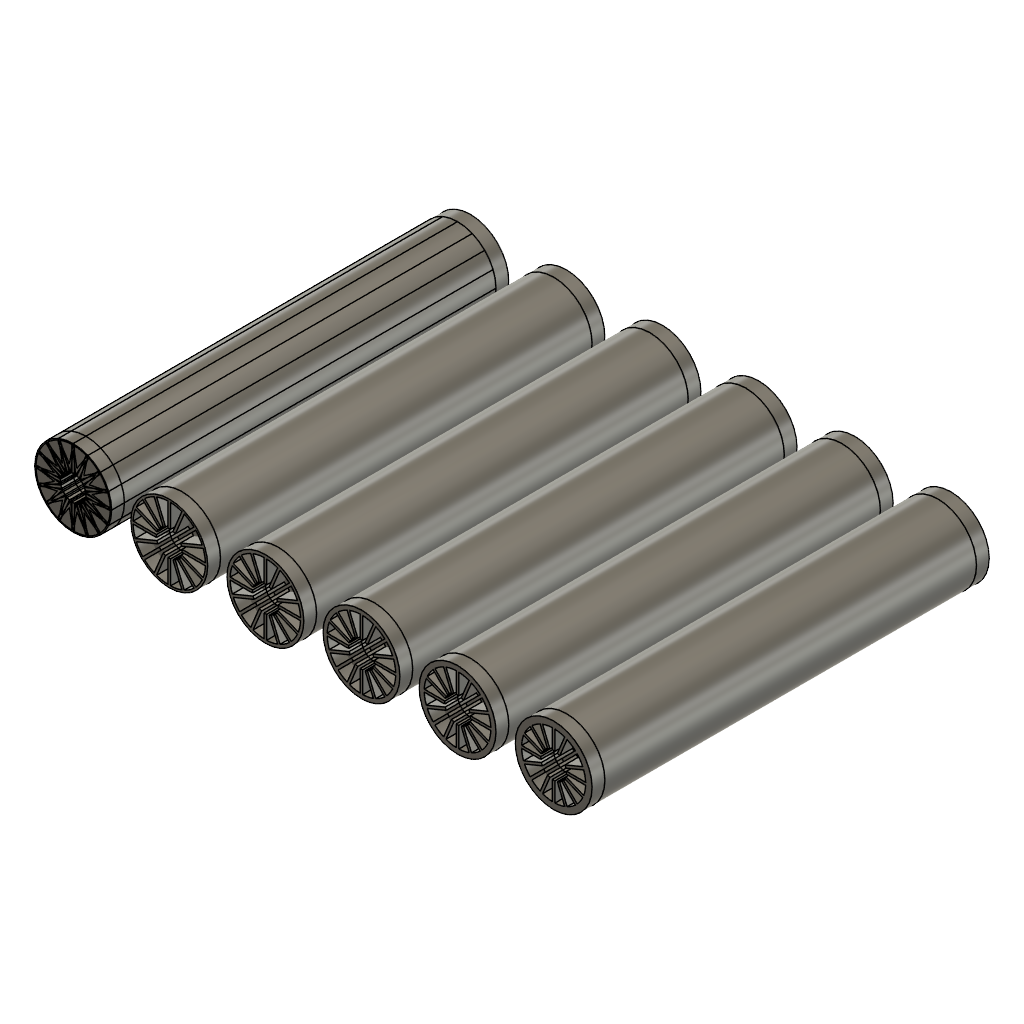
PAMcIA (Autodesk Fusion 360 design; units mm, degrees)
part number: 2026-09-20-16-45-00-598
Autodesk Fusion 360 part; units mm, degrees
sketch "Boceto1" plane through (0, 0, 0) normal (0, 0, 1) x (1, 0, 0)
  line L0 (6, 0) -> (2.9424, 0.5853)
  line L1 (2.9424, 0.5853) -> (5.5433, 2.2961)
  line L2 (5.5433, 2.2961) -> (2.4944, 1.6667)
  line L3 (2.4944, 1.6667) -> (4.2426, 4.2426)
  line L4 (4.2426, 4.2426) -> (1.6667, 2.4944)
  line L5 (1.6667, 2.4944) -> (2.2961, 5.5433)
  line L6 (2.2961, 5.5433) -> (0.5853, 2.9424)
  line L7 (0.5853, 2.9424) -> (0, 6)
  line L8 (0, 6) -> (-0.5853, 2.9424)
  line L9 (-0.5853, 2.9424) -> (-2.2961, 5.5433)
  line L10 (-2.2961, 5.5433) -> (-1.6667, 2.4944)
  line L11 (-1.6667, 2.4944) -> (-4.2426, 4.2426)
  line L12 (-4.2426, 4.2426) -> (-2.4944, 1.6667)
  line L13 (-2.4944, 1.6667) -> (-5.5433, 2.2961)
  line L14 (-5.5433, 2.2961) -> (-2.9424, 0.5853)
  line L15 (-2.9424, 0.5853) -> (-6, 0)
  line L16 (-6, 0) -> (-2.9424, -0.5853)
  line L17 (-2.9424, -0.5853) -> (-5.5433, -2.2961)
  line L18 (-5.5433, -2.2961) -> (-2.4944, -1.6667)
  line L19 (-2.4944, -1.6667) -> (-4.2426, -4.2426)
  line L20 (-4.2426, -4.2426) -> (-1.6667, -2.4944)
  line L21 (-1.6667, -2.4944) -> (-2.2961, -5.5433)
  line L22 (-2.2961, -5.5433) -> (-0.5853, -2.9424)
  line L23 (-0.5853, -2.9424) -> (0, -6)
  line L24 (0, -6) -> (0.5853, -2.9424)
  line L25 (0.5853, -2.9424) -> (2.2961, -5.5433)
  line L26 (2.2961, -5.5433) -> (1.6667, -2.4944)
  line L27 (1.6667, -2.4944) -> (4.2426, -4.2426)
  line L28 (4.2426, -4.2426) -> (2.4944, -1.6667)
  line L29 (2.4944, -1.6667) -> (5.5433, -2.2961)
  line L30 (5.5433, -2.2961) -> (2.9424, -0.5853)
  line L31 (2.9424, -0.5853) -> (6, 0)
  circle A0 centre (0, 0) radius 2
extrude "Extruir1" add sketch "Boceto1" along normal blind 60 makes body 1
sketch "Boceto2" plane through (0, 0, 0) normal (0, 0, 1) x (1, 0, 0)
  circle A0 centre (0, 0) radius 6
  line L0 (5, 0) -> (1.9616, 0.3902)
  line L1 (1.9616, 0.3902) -> (4.6194, 1.9134)
  line L2 (4.6194, 1.9134) -> (1.6629, 1.1111)
  line L3 (1.6629, 1.1111) -> (3.5355, 3.5355)
  line L4 (3.5355, 3.5355) -> (1.1111, 1.6629)
  line L5 (1.1111, 1.6629) -> (1.9134, 4.6194)
  line L6 (1.9134, 4.6194) -> (0.3902, 1.9616)
  line L7 (0.3902, 1.9616) -> (0, 5)
  line L8 (0, 5) -> (-0.3902, 1.9616)
  line L9 (-0.3902, 1.9616) -> (-1.9134, 4.6194)
  line L10 (-1.9134, 4.6194) -> (-1.1111, 1.6629)
  line L11 (-1.1111, 1.6629) -> (-3.5355, 3.5355)
  line L12 (-3.5355, 3.5355) -> (-1.6629, 1.1111)
  line L13 (-1.6629, 1.1111) -> (-4.6194, 1.9134)
  line L14 (-4.6194, 1.9134) -> (-1.9616, 0.3902)
  line L15 (-1.9616, 0.3902) -> (-5, 0)
  line L16 (-5, 0) -> (-1.9616, -0.3902)
  line L17 (-1.9616, -0.3902) -> (-4.6194, -1.9134)
  line L18 (-4.6194, -1.9134) -> (-1.6629, -1.1111)
  line L19 (-1.6629, -1.1111) -> (-3.5355, -3.5355)
  line L20 (-3.5355, -3.5355) -> (-1.1111, -1.6629)
  line L21 (-1.1111, -1.6629) -> (-1.9134, -4.6194)
  line L22 (-1.9134, -4.6194) -> (-0.3902, -1.9616)
  line L23 (-0.3902, -1.9616) -> (0, -5)
  line L24 (0, -5) -> (0.3902, -1.9616)
  line L25 (0.3902, -1.9616) -> (1.9134, -4.6194)
  line L26 (1.9134, -4.6194) -> (1.1111, -1.6629)
  line L27 (1.1111, -1.6629) -> (3.5355, -3.5355)
  line L28 (3.5355, -3.5355) -> (1.6629, -1.1111)
  line L29 (1.6629, -1.1111) -> (4.6194, -1.9134)
  line L30 (4.6194, -1.9134) -> (1.9616, -0.3902)
  line L31 (1.9616, -0.3902) -> (5, 0)
extrude "Extruir2" add sketch "Boceto2" along normal blind 60 separate body makes body 2
sketch "Boceto3" plane through (0, 0, 0) normal (0, 0, 1) x (1, 0, 0)
  circle A0 centre (0, 0) radius 6
  circle A1 centre (0, 0) radius 5.8
extrude "Extruir3" add sketch "Boceto3" along normal blind 60 separate body makes body 3
sketch "Boceto4" plane through (0, 0, 0) normal (0, 0, 1) x (1, 0, 0)
  line L0 (2, -0.2) -> (5.8, -0.2)
  line L1 (5.8, -0.2) -> (5.8, 0.2)
  line L2 (5.8, 0.2) -> (2, 0.2)
  line L3 (2, 0.2) -> (2, -0.2)
extrude "Extruir4" add sketch "Boceto4" along normal blind 60 separate body makes body 4
pattern_circular "Patrón C1" count 16 over 360 about axis through (0, 0, 1.75) along (0, 0, 1) of bodies 4 makes body 5 at (4.1117, 1.9196, 20) makes body 6 at (3.0641, 3.347, 20) makes body 7 at (1.5501, 4.2648, 20) makes body 8 at (-0.2, 4.5333, 20) makes body 9 at (-1.9196, 4.1117, 20) makes body 10 at (-3.347, 3.0641, 20) makes body 11 at (-4.2648, 1.5501, 20) makes body 12 at (-4.5333, -0.2, 20) makes body 13 at (-4.1117, -1.9196, 20) makes body 14 at (-3.0641, -3.347, 20) makes body 15 at (-1.5501, -4.2648, 20) makes body 16 at (0.2, -4.5333, 20) makes body 17 at (1.9196, -4.1117, 20) makes body 18 at (3.347, -3.0641, 20) makes body 19 at (4.2648, -1.5501, 20)
combine "Combinar1" operation add target body 3 tool bodies 4 5 6 7 8 9 10 11 12 13 14 15 16 17 18 19 4
sketch "Boceto5" plane through (0, 0, 0) normal (0, 0, 1) x (1, 0, 0)
  circle A0 centre (0, 0) radius 6
  circle A1 centre (0, 0) radius 5.65
extrude "Extruir5" add sketch "Boceto5" along normal blind 60 separate body makes body 20
sketch "Boceto6" plane through (0, 0, 0) normal (0, 0, 1) x (1, 0, 0)
  line L0 (2, -0.2) -> (5.65, -0.2)
  line L1 (5.65, -0.2) -> (5.65, 0.2)
  line L2 (5.65, 0.2) -> (2, 0.2)
  line L3 (2, 0.2) -> (2, -0.2)
extrude "Extruir6" add sketch "Boceto6" along normal blind 60 separate body makes body 21
pattern_circular "Patrón C2" count 16 over 360 about axis through (0, 0, 1.75) along (0, 0, 1) of bodies 21 makes body 22 at (4.0193, 1.8813, 20) makes body 23 at (2.9934, 3.2763, 20) makes body 24 at (1.5118, 4.1724, 20) makes body 25 at (-0.2, 4.4333, 40) makes body 26 at (-1.8813, 4.0193, 20) makes body 27 at (-3.2763, 2.9934, 40) makes body 28 at (-4.1724, 1.5118, 20) makes body 29 at (-4.4333, -0.2, 40) makes body 30 at (-4.0193, -1.8813, 20) makes body 31 at (-2.9934, -3.2763, 20) makes body 32 at (-1.5118, -4.1724, 20) makes body 33 at (0.2, -4.4333, 40) makes body 34 at (1.8813, -4.0193, 20) makes body 35 at (3.2763, -2.9934, 20) makes body 36 at (4.1724, -1.5118, 20)
combine "Combinar2" operation add target body 20 tool bodies 21 22 23 24 25 26 27 28 29 30 31 32 33 34 35 36 21
move_body "Desplazar1" bodies 20 to x (1, 0, 0) y (0, 1, 0) z (0, 0, 1) at (15, 0, 0)
sketch "Boceto7" plane through (0, 0, 0) normal (0, 0, 1) x (1, 0, 0)
  circle A0 centre (0, 0) radius 6
  circle A1 centre (0, 0) radius 5.5
extrude "Extruir7" add sketch "Boceto7" along normal blind 60 separate body makes body 37
sketch "Boceto8" plane through (0, 0, 0) normal (0, 0, 1) x (1, 0, 0)
  line L0 (2, -0.2) -> (5.5, -0.2)
  line L1 (5.5, -0.2) -> (5.5, 0.2)
  line L2 (5.5, 0.2) -> (2, 0.2)
  line L3 (2, 0.2) -> (2, -0.2)
extrude "Extruir8" add sketch "Boceto8" along normal blind 60 separate body makes body 38
pattern_circular "Patrón C3" count 16 over 360 about axis through (0, 0, 1.75) along (0, 0, 1) of bodies 38 makes body 39 at (3.9269, 1.8431, 20) makes body 40 at (2.9227, 3.2056, 20) makes body 41 at (1.4735, 4.08, 20) makes body 42 at (-0.2, 4.3333, 20) makes body 43 at (-1.8431, 3.9269, 20) makes body 44 at (-3.2056, 2.9227, 20) makes body 45 at (-4.08, 1.4735, 20) makes body 46 at (-4.3333, -0.2, 20) makes body 47 at (-3.9269, -1.8431, 20) makes body 48 at (-2.9227, -3.2056, 20) makes body 49 at (-1.4735, -4.08, 20) makes body 50 at (0.2, -4.3333, 20) makes body 51 at (1.8431, -3.9269, 20) makes body 52 at (3.2056, -2.9227, 20) makes body 53 at (4.08, -1.4735, 20)
combine "Combinar3" operation add target body 37 tool bodies 38 39 40 41 42 43 44 45 46 47 48 49 50 51 52 53 38
move_body "Desplazar2" bodies 37 to x (1, 0, 0) y (0, 1, 0) z (0, 0, 1) at (30, 0, 0)
sketch "Boceto9" plane through (0, 0, 0) normal (0, 0, 1) x (1, 0, 0)
  circle A0 centre (0, 0) radius 6
  circle A1 centre (0, 0) radius 5.35
extrude "Extruir9" add sketch "Boceto9" along normal blind 60 separate body makes body 54
sketch "Boceto10" plane through (0, 0, 0) normal (0, 0, 1) x (1, 0, 0)
  line L0 (2, -0.2) -> (5.35, -0.2)
  line L1 (5.35, -0.2) -> (5.35, 0.2)
  line L2 (5.35, 0.2) -> (2, 0.2)
  line L3 (2, 0.2) -> (2, -0.2)
extrude "Extruir10" add sketch "Boceto10" along normal blind 60 separate body makes body 55
pattern_circular "Patrón C4" count 16 over 360 about axis through (0, 0, 1.75) along (0, 0, 1) of bodies 55 makes body 56 at (2.956, 1.0079, 20) makes body 57 at (2.3452, 2.0624, 20) makes body 58 at (1.3775, 2.8029, 20) makes body 59 at (0.2, 3.1167, 20) makes body 60 at (-1.8048, 3.8346, 20) makes body 61 at (-3.1348, 2.852, 20) makes body 62 at (-3.9876, 1.4353, 20) makes body 63 at (-3.1167, 0.2, 20) makes body 64 at (-2.956, -1.0079, 20) makes body 65 at (-2.852, -3.1348, 20) makes body 66 at (-1.4353, -3.9876, 20) makes body 67 at (-0.2, -3.1167, 20) makes body 68 at (1.8048, -3.8346, 20) makes body 69 at (2.0624, -2.3452, 20) makes body 70 at (3.9876, -1.4353, 20)
combine "Combinar4" operation add target body 54 tool bodies 55 56 57 58 59 60 61 62 63 64 65 66 67 68 69 70 55
move_body "Desplazar3" bodies 54 to x (1, 0, 0) y (0, 1, 0) z (0, 0, 1) at (45, 0, 0)
sketch "Boceto11" plane through (0, 0, 0) normal (0, 0, 1) x (1, 0, 0)
  circle A0 centre (0, 0) radius 6
  circle A1 centre (0, 0) radius 5.2
extrude "Extruir11" add sketch "Boceto11" along normal blind 60 separate body makes body 71
sketch "Boceto12" plane through (0, 0, 0) normal (0, 0, 1) x (1, 0, 0)
  line L0 (2, -0.2) -> (5.2, -0.2)
  line L1 (5.2, -0.2) -> (5.2, 0.2)
  line L2 (5.2, 0.2) -> (2, 0.2)
  line L3 (2, 0.2) -> (2, -0.2)
extrude "Extruir12" add sketch "Boceto12" along normal blind 60 separate body makes body 72
pattern_circular "Patrón C5" count 16 over 360 about axis through (0, 0, 1.75) along (0, 0, 1) of bodies 72 makes body 73 at (3.7422, 1.7665, 20) makes body 74 at (2.7813, 3.0641, 20) makes body 75 at (1.397, 3.8952, 20) makes body 76 at (-0.2, 4.1333, 20) makes body 77 at (-1.7665, 3.7422, 20) makes body 78 at (-3.0641, 2.7813, 20) makes body 79 at (-3.8952, 1.397, 20) makes body 80 at (-4.1333, -0.2, 20) makes body 81 at (-3.7422, -1.7665, 20) makes body 82 at (-2.7813, -3.0641, 20) makes body 83 at (-1.397, -3.8952, 20) makes body 84 at (0.2, -4.1333, 20) makes body 85 at (1.7665, -3.7422, 20) makes body 86 at (3.0641, -2.7813, 20) makes body 87 at (3.8952, -1.397, 20)
combine "Combinar5" operation add target body 71 tool bodies 72 73 74 75 76 77 78 79 80 81 82 83 84 85 86 87 72
move_body "Desplazar4" bodies 71 to x (1, 0, 0) y (0, 1, 0) z (0, 0, 1) at (60, 0, 0)
sketch "Boceto13" plane through (0, 0, 0) normal (0, 0, 1) x (1, 0, 0)
  circle A0 centre (0, 0) radius 6
  circle A1 centre (0, 0) radius 5
extrude "Extruir13" add sketch "Boceto13" along normal blind 60 separate body makes body 88
sketch "Boceto14" plane through (0, 0, 0) normal (0, 0, 1) x (1, 0, 0)
  line L0 (2, -0.2) -> (5, -0.2)
  line L1 (5, -0.2) -> (5, 0.2)
  line L2 (5, 0.2) -> (2, 0.2)
  line L3 (2, 0.2) -> (2, -0.2)
extrude "Extruir14" add sketch "Boceto14" along normal blind 60 separate body makes body 89
pattern_circular "Patrón C6" count 16 over 360 about axis through (0, 0, 1.75) along (0, 0, 1) of bodies 89 makes body 90 at (3.619, 1.7155, 20) makes body 91 at (2.687, 2.9698, 20) makes body 92 at (1.346, 3.7721, 20) makes body 93 at (-0.2, 4, 20) makes body 94 at (-1.7155, 3.619, 20) makes body 95 at (-2.9698, 2.687, 20) makes body 96 at (-3.7721, 1.346, 20) makes body 97 at (-4, -0.2, 20) makes body 98 at (-3.619, -1.7155, 20) makes body 99 at (-2.687, -2.9698, 20) makes body 100 at (-1.346, -3.7721, 20) makes body 101 at (0.2, -4, 20) makes body 102 at (1.7155, -3.619, 20) makes body 103 at (2.9698, -2.687, 20) makes body 104 at (3.7721, -1.346, 20)
combine "Combinar6" operation add target body 88 tool bodies 89 90 91 92 93 94 95 96 97 98 99 100 101 102 103 104 89
move_body "Desplazar5" bodies 88 to x (1, 0, 0) y (0, 1, 0) z (0, 0, 1) at (75, 0, 0)
sketch "Boceto15" plane through (0, 0, 0) normal (0, 0, 1) x (1, 0, 0)
  circle A0 centre (0, 0) radius 6
extrude "Extruir15" add sketch "Boceto15" against normal blind 2 separate body makes body 105
sketch "Boceto16" plane through (0, 0, 0) normal (0, 0, 1) x (1, 0, 0)
  circle A0 centre (0, 0) radius 6
  circle A1 centre (0, 0) radius 5.8
extrude "Extruir16" add sketch "Boceto16" along normal blind 48 separate body makes body 106
sketch "Boceto17" plane through (0, 0, 0) normal (0, 0, 1) x (1, 0, 0)
  line L0 (2, -0.2) -> (5.8, -0.2)
  line L1 (5.8, -0.2) -> (5.8, 0.2)
  line L2 (5.8, 0.2) -> (2, 0.2)
  line L3 (2, 0.2) -> (2, -0.2)
extrude "Extruir17" add sketch "Boceto17" along normal blind 48 separate body makes body 107
pattern_circular "Patrón C7" count 16 over 360 about axis through (0, 0, 1.75) along (0, 0, 1) of bodies 107 makes body 108 at (4.1117, 1.9196, 16) makes body 109 at (3.0641, 3.347, 16) makes body 110 at (1.5501, 4.2648, 16) makes body 111 at (-0.2, 4.5333, 16) makes body 112 at (-1.9196, 4.1117, 16) makes body 113 at (-3.347, 3.0641, 16) makes body 114 at (-4.2648, 1.5501, 16) makes body 115 at (-4.5333, -0.2, 16) makes body 116 at (-4.1117, -1.9196, 16) makes body 117 at (-3.0641, -3.347, 16) makes body 118 at (-1.5501, -4.2648, 16) makes body 119 at (0.2, -4.5333, 16) makes body 120 at (1.9196, -4.1117, 16) makes body 121 at (3.347, -3.0641, 16) makes body 122 at (4.2648, -1.5501, 16)
sketch "Boceto18" plane through (0, 0, 0) normal (0, 0, 1) x (1, 0, 0)
  circle A0 centre (0, 0) radius 6
  circle A1 centre (0, 0) radius 2
extrude "Extruir18" add sketch "Boceto18" along normal blind 10 separate body makes body 123
move_body "Desplazar6" bodies 123 to x (1, 0, 0) y (0, 1, 0) z (0, 0, 1) at (0, 0, 48)
combine "Combinar7" operation add target body 106 tool bodies 105 123 107 108 109 110 111 112 113 114 115 116 117 118 119 120 121 122 107
sketch "Boceto19" plane through (0, 0, 0) normal (0, 0, 1) x (1, 0, 0)
  circle A0 centre (0, 0) radius 6
extrude "Extruir19" add sketch "Boceto19" against normal blind 2 separate body makes body 124
sketch "Boceto20" plane through (0, 0, 0) normal (0, 0, 1) x (1, 0, 0)
  circle A0 centre (0, 0) radius 6
  circle A1 centre (0, 0) radius 5.65
extrude "Extruir20" add sketch "Boceto20" along normal blind 48 separate body makes body 125
sketch "Boceto21" plane through (0, 0, 0) normal (0, 0, 1) x (1, 0, 0)
  line L0 (2, -0.2) -> (5.65, -0.2)
  line L1 (5.65, -0.2) -> (5.65, 0.2)
  line L2 (5.65, 0.2) -> (2, 0.2)
  line L3 (2, 0.2) -> (2, -0.2)
extrude "Extruir21" add sketch "Boceto21" along normal blind 48 separate body makes body 126
pattern_circular "Patrón C8" count 16 over 360 about axis through (0, 0, 1.75) along (0, 0, 1) of bodies 126 makes body 127 at (4.0193, 1.8813, 16) makes body 128 at (2.9934, 3.2763, 16) makes body 129 at (1.5118, 4.1724, 16) makes body 130 at (-0.2, 4.4333, 32) makes body 131 at (-1.8813, 4.0193, 16) makes body 132 at (-3.2763, 2.9934, 16) makes body 133 at (-4.1724, 1.5118, 16) makes body 134 at (-4.4333, -0.2, 32) makes body 135 at (-4.0193, -1.8813, 16) makes body 136 at (-2.9934, -3.2763, 16) makes body 137 at (-1.5118, -4.1724, 16) makes body 138 at (0.2, -4.4333, 32) makes body 139 at (1.8813, -4.0193, 16) makes body 140 at (3.2763, -2.9934, 16) makes body 141 at (4.1724, -1.5118, 16)
sketch "Boceto22" plane through (0, 0, 0) normal (0, 0, 1) x (1, 0, 0)
  circle A0 centre (0, 0) radius 6
  circle A1 centre (0, 0) radius 2
extrude "Extruir22" add sketch "Boceto22" along normal blind 10 separate body makes body 142
move_body "Desplazar7" bodies 142 to x (1, 0, 0) y (0, 1, 0) z (0, 0, 1) at (0, 0, 48)
combine "Combinar8" operation add target body 125 tool bodies 124 142 126 127 128 129 130 131 132 133 134 135 136 137 138 139 140 141 126
move_body "Desplazar8" bodies 125 to x (1, 0, 0) y (0, 1, 0) z (0, 0, 1) at (15, 0, 0)
sketch "Boceto23" plane through (0, 0, 0) normal (0, 0, 1) x (1, 0, 0)
  circle A0 centre (0, 0) radius 6
extrude "Extruir23" add sketch "Boceto23" against normal blind 2 separate body makes body 143
sketch "Boceto24" plane through (0, 0, 0) normal (0, 0, 1) x (1, 0, 0)
  circle A0 centre (0, 0) radius 6
  circle A1 centre (0, 0) radius 5.5
extrude "Extruir24" add sketch "Boceto24" along normal blind 48 separate body makes body 144
sketch "Boceto25" plane through (0, 0, 0) normal (0, 0, 1) x (1, 0, 0)
  line L0 (2, -0.2) -> (5.5, -0.2)
  line L1 (5.5, -0.2) -> (5.5, 0.2)
  line L2 (5.5, 0.2) -> (2, 0.2)
  line L3 (2, 0.2) -> (2, -0.2)
extrude "Extruir25" add sketch "Boceto25" along normal blind 48 separate body makes body 145
pattern_circular "Patrón C9" count 16 over 360 about axis through (0, 0, 1.75) along (0, 0, 1) of bodies 145 makes body 146 at (3.9269, 1.8431, 16) makes body 147 at (2.9227, 3.2056, 16) makes body 148 at (1.4735, 4.08, 16) makes body 149 at (-0.2, 4.3333, 16) makes body 150 at (-1.8431, 3.9269, 16) makes body 151 at (-3.2056, 2.9227, 16) makes body 152 at (-4.08, 1.4735, 16) makes body 153 at (-4.3333, -0.2, 16) makes body 154 at (-3.9269, -1.8431, 16) makes body 155 at (-2.9227, -3.2056, 32) makes body 156 at (-1.4735, -4.08, 16) makes body 157 at (0.2, -4.3333, 16) makes body 158 at (1.8431, -3.9269, 16) makes body 159 at (3.2056, -2.9227, 16) makes body 160 at (4.08, -1.4735, 16)
sketch "Boceto26" plane through (0, 0, 0) normal (0, 0, 1) x (1, 0, 0)
  circle A0 centre (0, 0) radius 6
  circle A1 centre (0, 0) radius 2
extrude "Extruir26" add sketch "Boceto26" along normal blind 10 separate body makes body 161
move_body "Desplazar9" bodies 161 to x (1, 0, 0) y (0, 1, 0) z (0, 0, 1) at (0, 0, 48)
combine "Combinar9" operation add target body 144 tool bodies 143 161 145 146 147 148 149 150 151 152 153 154 155 156 157 158 159 160 145
move_body "Desplazar10" bodies 144 to x (1, 0, 0) y (0, 1, 0) z (0, 0, 1) at (30, 0, 0)
sketch "Boceto27" plane through (0, 0, 0) normal (0, 0, 1) x (1, 0, 0)
  circle A0 centre (0, 0) radius 6
extrude "Extruir27" add sketch "Boceto27" against normal blind 2 separate body makes body 162
sketch "Boceto28" plane through (0, 0, 0) normal (0, 0, 1) x (1, 0, 0)
  circle A0 centre (0, 0) radius 6
  circle A1 centre (0, 0) radius 5.35
extrude "Extruir28" add sketch "Boceto28" along normal blind 48 separate body makes body 163
sketch "Boceto29" plane through (0, 0, 0) normal (0, 0, 1) x (1, 0, 0)
  line L0 (2, -0.2) -> (5.35, -0.2)
  line L1 (5.35, -0.2) -> (5.35, 0.2)
  line L2 (5.35, 0.2) -> (2, 0.2)
  line L3 (2, 0.2) -> (2, -0.2)
extrude "Extruir29" add sketch "Boceto29" along normal blind 48 separate body makes body 164
pattern_circular "Patrón C10" count 16 over 360 about axis through (0, 0, 1.75) along (0, 0, 1) of bodies 164 makes body 165 at (2.956, 1.0079, 16) makes body 166 at (2.3452, 2.0624, 16) makes body 167 at (1.3775, 2.8029, 16) makes body 168 at (0.2, 3.1167, 16) makes body 169 at (-1.8048, 3.8346, 16) makes body 170 at (-3.1348, 2.852, 16) makes body 171 at (-3.9876, 1.4353, 16) makes body 172 at (-3.1167, 0.2, 16) makes body 173 at (-2.956, -1.0079, 16) makes body 174 at (-2.852, -3.1348, 16) makes body 175 at (-1.4353, -3.9876, 16) makes body 176 at (-0.2, -3.1167, 16) makes body 177 at (1.8048, -3.8346, 16) makes body 178 at (2.0624, -2.3452, 16) makes body 179 at (3.9876, -1.4353, 16)
sketch "Boceto30" plane through (0, 0, 0) normal (0, 0, 1) x (1, 0, 0)
  circle A0 centre (0, 0) radius 6
  circle A1 centre (0, 0) radius 2
extrude "Extruir30" add sketch "Boceto30" along normal blind 10 separate body makes body 180
move_body "Desplazar11" bodies 180 to x (1, 0, 0) y (0, 1, 0) z (0, 0, 1) at (0, 0, 48)
combine "Combinar10" operation add target body 163 tool bodies 162 180 164 165 166 167 168 169 170 171 172 173 174 175 176 177 178 179 164
move_body "Desplazar12" bodies 163 to x (1, 0, 0) y (0, 1, 0) z (0, 0, 1) at (45, 0, 0)
sketch "Boceto31" plane through (0, 0, 0) normal (0, 0, 1) x (1, 0, 0)
  circle A0 centre (0, 0) radius 6
extrude "Extruir31" add sketch "Boceto31" against normal blind 2 separate body makes body 181
sketch "Boceto32" plane through (0, 0, 0) normal (0, 0, 1) x (1, 0, 0)
  circle A0 centre (0, 0) radius 6
  circle A1 centre (0, 0) radius 5.2
extrude "Extruir32" add sketch "Boceto32" along normal blind 48 separate body makes body 182
sketch "Boceto33" plane through (0, 0, 0) normal (0, 0, 1) x (1, 0, 0)
  line L0 (2, -0.2) -> (5.2, -0.2)
  line L1 (5.2, -0.2) -> (5.2, 0.2)
  line L2 (5.2, 0.2) -> (2, 0.2)
  line L3 (2, 0.2) -> (2, -0.2)
extrude "Extruir33" add sketch "Boceto33" along normal blind 48 separate body makes body 183
pattern_circular "Patrón C11" count 16 over 360 about axis through (0, 0, 1.75) along (0, 0, 1) of bodies 183 makes body 184 at (3.7422, 1.7665, 32) makes body 185 at (2.7813, 3.0641, 16) makes body 186 at (1.397, 3.8952, 32) makes body 187 at (-0.2, 4.1333, 32) makes body 188 at (-1.7665, 3.7422, 16) makes body 189 at (-3.0641, 2.7813, 16) makes body 190 at (-3.8952, 1.397, 16) makes body 191 at (-4.1333, -0.2, 32) makes body 192 at (-3.7422, -1.7665, 16) makes body 193 at (-2.7813, -3.0641, 32) makes body 194 at (-1.397, -3.8952, 16) makes body 195 at (0.2, -4.1333, 32) makes body 196 at (1.7665, -3.7422, 32) makes body 197 at (3.0641, -2.7813, 16) makes body 198 at (3.8952, -1.397, 16)
sketch "Boceto34" plane through (0, 0, 0) normal (0, 0, 1) x (1, 0, 0)
  circle A0 centre (0, 0) radius 6
  circle A1 centre (0, 0) radius 2
extrude "Extruir34" add sketch "Boceto34" along normal blind 10 separate body makes body 199
move_body "Desplazar13" bodies 199 to x (1, 0, 0) y (0, 1, 0) z (0, 0, 1) at (0, 0, 48)
combine "Combinar11" operation add target body 182 tool bodies 181 199 183 184 185 186 187 188 189 190 191 192 193 194 195 196 197 198 183
move_body "Desplazar14" bodies 182 to x (1, 0, 0) y (0, 1, 0) z (0, 0, 1) at (60, 0, 0)
sketch "Boceto35" plane through (0, 0, 0) normal (0, 0, 1) x (1, 0, 0)
  circle A0 centre (0, 0) radius 6
extrude "Extruir35" add sketch "Boceto35" against normal blind 2 separate body makes body 200
sketch "Boceto36" plane through (0, 0, 0) normal (0, 0, 1) x (1, 0, 0)
  circle A0 centre (0, 0) radius 6
  circle A1 centre (0, 0) radius 5
extrude "Extruir36" add sketch "Boceto36" along normal blind 48 separate body makes body 201
sketch "Boceto37" plane through (0, 0, 0) normal (0, 0, 1) x (1, 0, 0)
  line L0 (2, -0.2) -> (5, -0.2)
  line L1 (5, -0.2) -> (5, 0.2)
  line L2 (5, 0.2) -> (2, 0.2)
  line L3 (2, 0.2) -> (2, -0.2)
extrude "Extruir37" add sketch "Boceto37" along normal blind 48 separate body makes body 202
pattern_circular "Patrón C12" count 16 over 360 about axis through (0, 0, 1.75) along (0, 0, 1) of bodies 202 makes body 203 at (3.619, 1.7155, 16) makes body 204 at (2.687, 2.9698, 16) makes body 205 at (1.346, 3.7721, 16) makes body 206 at (-0.2, 4, 16) makes body 207 at (-1.7155, 3.619, 16) makes body 208 at (-2.9698, 2.687, 16) makes body 209 at (-3.7721, 1.346, 16) makes body 210 at (-4, -0.2, 16) makes body 211 at (-3.619, -1.7155, 16) makes body 212 at (-2.687, -2.9698, 16) makes body 213 at (-1.346, -3.7721, 16) makes body 214 at (0.2, -4, 16) makes body 215 at (1.7155, -3.619, 16) makes body 216 at (2.9698, -2.687, 16) makes body 217 at (3.7721, -1.346, 16)
sketch "Boceto38" plane through (0, 0, 0) normal (0, 0, 1) x (1, 0, 0)
  circle A0 centre (0, 0) radius 6
  circle A1 centre (0, 0) radius 2
extrude "Extruir38" add sketch "Boceto38" along normal blind 10 separate body makes body 218
move_body "Desplazar15" bodies 218 to x (1, 0, 0) y (0, 1, 0) z (0, 0, 1) at (0, 0, 48)
combine "Combinar12" operation add target body 201 tool bodies 200 218 202 203 204 205 206 207 208 209 210 211 212 213 214 215 216 217 202
move_body "Desplazar16" bodies 201 to x (1, 0, 0) y (0, 1, 0) z (0, 0, 1) at (75, 0, 0)
